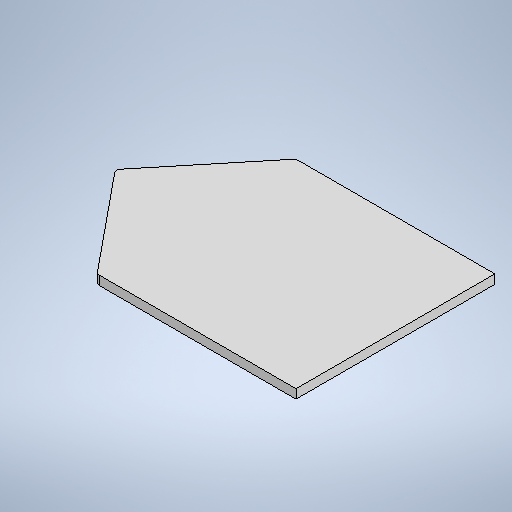
# Autodesk Inventor part: MNT-CDF-604 CAP
Saved by Autodesk Inventor 2025 (Build 290162010, 162A)
## iProperties
Created: 2025-01-16
Part Number: MNT-CDF-604 CAP
Material: Stainless Steel
Document SubType Name: Sheet Metal
Designer: pokla
Density: 8 g/cm^3
Sheet Metal Rule: AISI304 2mm Die16
Appearance: Default
Author: pokla
Autodesk Inventor part; units mm, degrees
ref_plane "YZ Plane" through (0, 0, 0) normal (1, 0, 0) x (0, 1, 0)
ref_plane "XZ Plane" through (0, 0, 0) normal (0, 1, 0) x (-1, 0, 0)
ref_plane "XY Plane" through (0, 0, 0) normal (0, 0, 1) x (1, 0, 0)
sketch "Sketch1" plane through (0, 0, 0) normal (0, 0, 1) x (1, 0, 0)
  line L0 (-22, 22) -> (22, 22)
  line L1 (22, 22) -> (22, -22)
  line L2 (22, -22) -> (-22, -22)
  line L3 (-22, -22) -> (-22, 22) construction
  line L4 (-22, 22) -> (22, -22) construction
  line L5 (-22, -22) -> (-40, 0)
  line L6 (-40, 0) -> (-22, 22)
  point P0 (0, 0)
  point P1 (0, 0)
  point P2 (22, 0)
  dimension "d0" = 44
  dimension "d1" = 44
  dimension "d4" = 62
  measures "d0" distance of L0.start L0.end
  measures "d1" distance of L2.end L0.start
  measures "d4" distance of point (22, 0) L5.end
extrude "Plate1" add sketch "Sketch1" along normal blind 2
fillet "Corner Round2" radius 1 3 edges at (-22, -22, 1) (-40, 0, 1) (-22, 22, 1)
equation "\"d2\" = Thickness"
equation "\"BendReliefWidth\" = Thickness"
equation "\"BendReliefDepth\" = 0.5 * Thickness"
equation "\"CornerReliefSize\" = 4 * Thickness"
equation "\"MinimumRemnant\" = 2 * Thickness"
equation "\"TransitionRadius\" = BendRadius"
equation "\"JacobiRadiusSize\" = BendRadius"
equation "\"GapSize\" = Thickness"
equation "\"Thickness\" = 2"
equation "\"BendRadius\" = 2.75"
body "Solid1"
